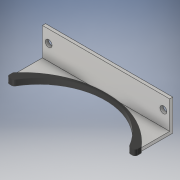
# Autodesk Inventor part: Glashalter
Saved by Autodesk Inventor 2019 (Build 230136000, 136)
## iProperties
Created: 2019-02-21
Part Number: Glashalter
Material: Generisch
Document SubType Name: Modeling
Designer: nico-
Density: 1 g/cm^3
Appearance: Vorgabe
Author: nico-
Autodesk Inventor part; units mm, degrees
ref_plane "YZ Plane" through (0, 0, 0) normal (1, 0, 0) x (0, 1, 0)
ref_plane "XZ Plane" through (0, 0, 0) normal (0, 1, 0) x (-1, 0, 0)
ref_plane "XY Plane" through (0, 0, 0) normal (0, 0, 1) x (1, 0, 0)
sketch "Skizze1" plane through (0, 0, 0) normal (1, 0, 0) x (0, 1, 0)
  line L0 (0, 0) -> (0, -30)
  line L1 (0, -30) -> (25, -30)
  line L2 (25, -30) -> (25, -27.5)
  line L3 (25, -27.5) -> (2.5, -27.5)
  line L4 (2.5, -27.5) -> (2.5, 0)
  line L5 (2.5, 0) -> (0, 0)
  dimension "d0" = 30
  dimension "d1" = 25
  dimension "d2" = 2.5
  dimension "d3" = 22.5
  constraints: 12 end point, 5 perpendicular, 1 vertical
  measures "d0" distance of L0.start L0.end
  measures "d1" distance of L0.end L1.end
  measures "d2" distance of L1.end L2.end
  measures "d3" distance of L2.end L3.end
extrude "Extrusion1" add sketch "Skizze1" along normal mid plane 102
sketch "Skizze2" plane through (-51, 2.5, 0) normal (0, 1, 0) x (1, 0, 0)
  line L0 (0, 0) -> (102, 0) projected
  arc A0 (98, 0) -> (4, 0) centre (51, -26.4136) ccw
  line L1 (0, 27.5) -> (102, 27.5) projected
  line L2 (4, 0) -> (98, 0)
  point P0 (51, 0)
  dimension "d6" = 94
  constraints: 2 end point, 2 point on circle, 2 point on line, 1 centre point, 1 collinear, 1 tangent
  measures "d6" distance of L2.start L2.end
extrude "Extrusion2" cut sketch "Skizze2" against normal blind 2.5
fillet "Rundung1" radius 2 4 edges at (-47, 1.25, 0) (-51, 1.25, 0) (47, 1.25, 0) (51, 1.25, 0)
sketch "Skizze3" plane through (-51, 2.5, -27.5) normal (0, 1, 0) x (1, 0, 0)
  line L0 (-0.5, 0) -> (27.5, 0) construction
  line L1 (-0.5, -28) -> (4.5665, -28)
  arc A0 (97.4335, -28) -> (4.5665, -28) centre (51, -53.8505) ccw
  line L2 (102.2546, -28) -> (97.4335, -28)
  line L3 (51, 0) -> (102, 0) projected
  line L4 (-0.5, -28) -> (-0.5, -23)
  arc A1 (51, 0) -> (-0.5, -23) centre (49.8083, -66.4893) ccw
  line L5 (102.2546, -28) -> (102.2546, -23)
  line L6 (102, 0) -> (102, -25.5) projected
  line L7 (102.2546, -28) -> (107.2546, -28) construction
  arc A2 (97.4335, -26.5163) -> (51, 0) centre (51, -53.9136) ccw projected
  arc A3 (102.2546, -23) -> (51, 0) centre (51.9496, -66.4932) ccw
  point P0 (51, -27.5)
  dimension "d10" = 28
  dimension "d13" = 5
  dimension "d14" = 66.5
  dimension "d20" = 5
  dimension "d21" = 90
  dimension "d22" = 66.5
  constraints: 12 end point, 6 point on circle, 3 centre point, 3 horizontal, 1 parallel, 1 perpendicular, 1 vertical
  measures "d10" distance of L0.start L1.start
  measures "d13" distance of L1.start L4.end
  measures "d14" radius of A1
  measures "d20" distance of L2.start L5.end
  measures "d21" angle of L7 L5
  measures "d22" radius of A3
extrude "Extrusion3" add sketch "Skizze3" along normal blind 1 and the other way blind 3.5 contours L4 A1 L3 A3 L5 L2 A0 L1 | A3 L3
fillet "Rundung2" radius 2 4 edges at (51.2546, 1.25, 0.5) (46.4335, 1.25, 0.5) (-46.4335, 1.25, 0.5) (-51.5, 1.25, 0.5)
sketch "Skizze4" plane through (-51, 25, -27.5) normal (0, 0, 1) x (1, 0, 0)
  circle A0 centre (97, -10) radius 2.75
  circle A1 centre (5, -10) radius 2.75
  point P0 (51, -25)
  dimension "d24" = 5.5
  dimension "d25" = 5.5
  constraints: 2 centre point
  measures "d24" diameter of A0
  measures "d25" diameter of A1
extrude "Extrusion4" cut sketch "Skizze4" against normal blind 2.5
